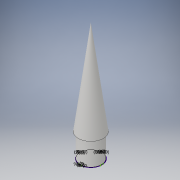
# Autodesk Inventor part: Nose Cone MK II [incomplete]
Saved by Autodesk Inventor 2017 (Build 210142000, 142)
## iProperties
Created: 2017-05-18
Part Number: Nose Cone MK II [incomplete]
Material: Generic
Document SubType Name: Modeling
Designer: Harrison
Density: 1 g/cm^3
Appearance: Default
Author: Harrison
Autodesk Inventor part; units mm, degrees
ref_plane "YZ Plane" through (0, 0, 0) normal (1, 0, 0) x (0, 1, 0)
ref_plane "XZ Plane" through (0, 0, 0) normal (0, 1, 0) x (-1, 0, 0)
ref_plane "XY Plane" through (0, 0, 0) normal (0, 0, 1) x (1, 0, 0)
sketch "Sketch1" plane through (0, 0, 0) normal (1, 0, 0) x (0, 1, 0)
  line L0 (0, 0) -> (101.6, 0)
  line L1 (0, -11.557) -> (0, -13.462)
  line L2 (0, -13.462) -> (101.6, 0)
  line L3 (0, 0) -> (-25.4, 0)
  line L4 (-25.4, 0) -> (-25.4, -11.557)
  line L5 (-25.4, -11.557) -> (0, -11.557)
  line L6 (1.27, -10.287) -> (1.27, -12.0126)
  line L7 (1.27, -12.0126) -> (82.3464, -1.27)
  line L8 (0, -10.287) -> (-24.13, -10.287)
  line L9 (82.3464, -1.27) -> (91.9313, 0)
  line L10 (0, -10.287) -> (1.27, -10.287)
  line L11 (-24.13, -10.287) -> (-25.4, -10.287)
  dimension "d0" = 101.6
  dimension "d1" = 13.462
  dimension "d2" = 25.4
  dimension "d3" = 11.557
  dimension "d4" = 1.27
  dimension "d5" = 1.27
  constraints: 24 end point, 3 perpendicular, 2 horizontal, 2 point on line, 2 vertical
  measures "d0" distance of L0.start L0.end
  measures "d1" distance of L0.start L1.end
  measures "d2" distance of L0.start L3.end
  measures "d3" distance of L3.end L4.end
  measures "d4" distance between parallel lines of L2 L7
  measures "d5" distance between parallel lines of L5 L8
revolve "Revolution1" add sketch "Sketch1" angle 360 about axis through (0, 0, 0) along (0, 1, 0) contours L0 L2 L1 L5 L4 L11 L8 L10 L6 L7 L9
sketch "Sketch2" plane through (0, -25.4, 0) normal (0, -1, 0) x (1, 0, 0)
  circle A0 centre (0, 0) radius 11.557
  circle A1 centre (0, 0) radius 11.811
  circle A2 centre (0, 0) radius 11.557 projected
  line L0 (-0.0952, -11.5566) -> (-1.6827, -11.5566)
  line L1 (-1.6827, -11.5566) -> (1.4923, -11.5566)
  line L2 (-1.6827, -11.5566) -> (1.4923, -11.5566) construction
  line L3 (0, 0) -> (-15.1978, 0)
  line L4 (-11.557, 0) -> (-11.557, -1.5875)
  line L5 (-11.557, 0) -> (-9.9695, 0) construction
  line L6 (-11.557, 0) -> (-11.557, 1.5875)
  line L7 (-0.0029, 11.557) -> (-1.5904, 11.557)
  line L8 (-0.0029, 11.557) -> (1.5846, 11.557)
  line L9 (11.557, -0.0003) -> (11.557, 1.5872)
  line L10 (11.557, -0.0003) -> (13.1445, -0.0003) construction
  line L11 (11.557, 1.5872) -> (11.557, -1.5806)
  line L12 (1.5846, 11.7042) -> (1.5846, 11.4479)
  line L13 (1.5846, 11.7042) -> (1.8409, 11.7042) construction
  line L14 (-1.5846, 11.7042) -> (-1.5846, 11.4479)
  line L15 (-1.5846, 11.7042) -> (-1.3282, 11.7042) construction
  line L16 (-11.4484, 1.5806) -> (-11.7048, 1.5806)
  line L17 (-11.7048, -1.5806) -> (-11.4474, -1.5882)
  line L18 (11.7048, -1.5806) -> (11.4484, -1.5806)
  circle A3 centre (0, 0) radius 11.557
  circle A4 centre (0, 0) radius 11.811
  line L19 (-11.7042, -1.5846) -> (-11.4479, -1.5846)
  line L20 (-11.7042, -1.5846) -> (-11.7042, -1.3282) construction
  line L21 (-11.557, -0.0029) -> (-11.557, -1.5904)
  line L22 (-11.557, -0.0029) -> (-11.557, 1.5846)
  line L23 (-11.7042, 1.5846) -> (-11.4479, 1.5846)
  line L24 (-11.7042, 1.5846) -> (-11.7042, 1.8409) construction
  circle A5 centre (0, 0) radius 11.557
  circle A6 centre (0, 0) radius 11.811
  line L25 (1.5846, -11.7042) -> (1.5846, -11.4479)
  line L26 (1.5846, -11.7042) -> (1.3282, -11.7042) construction
  line L27 (0.0029, -11.557) -> (1.5904, -11.557)
  line L28 (0.0029, -11.557) -> (-1.5846, -11.557)
  line L29 (-1.5846, -11.7042) -> (-1.5846, -11.4479)
  line L30 (-1.5846, -11.7042) -> (-1.8409, -11.7042) construction
  circle A7 centre (0, 0) radius 11.557
  circle A8 centre (0, 0) radius 11.811
  line L31 (11.7042, 1.5846) -> (11.4479, 1.5846)
  line L32 (11.7042, 1.5846) -> (11.7042, 1.3282) construction
  line L33 (11.557, 0.0029) -> (11.557, 1.5904)
  line L34 (11.557, 0.0029) -> (11.557, -1.5846)
  line L35 (11.7042, -1.5846) -> (11.4479, -1.5846)
  line L36 (11.7042, -1.5846) -> (11.7042, -1.8409) construction
  point P0 (11.5566, -0.0952)
  point P1 (0.0003, 11.557)
  point P2 (-1.5806, -11.4484)
  point P3 (1.5882, -11.4474)
  point P4 (-1.5806, -11.7048)
  point P5 (1.5806, -11.7048)
  point P6 (1.5806, 11.7048)
  point P7 (0.0952, 11.5566)
  point P8 (-11.557, 0.0003)
  point P9 (11.4484, -1.5806)
  point P10 (11.4474, 1.5882)
  point P11 (11.7048, -1.5806)
  point P12 (11.7048, 1.5806)
  point P13 (-11.7048, 1.5806)
  point P14 (-11.5566, 0.0952)
  point P15 (-0.0003, -11.557)
  point P16 (1.5806, 11.4484)
  point P17 (-1.5882, 11.4474)
  point P18 (1.5806, 11.7048)
  point P19 (-1.5806, 11.7048)
  point P20 (-1.5806, -11.7048)
  dimension "d7" = 0.254
  dimension "d8" = 1.5875
  dimension "d9" = 3.175
  dimension "d10" = 0
  dimension "d11" = 1.5875
  dimension "d12" = 90
  dimension "d13" = 1.5875
  dimension "d14" = 1.5875
  dimension "d15" = 1.5875
  dimension "d20" = 90
  dimension "d21" = 90
  dimension "d25" = 360
  constraints: 74 end point, 40 point on circle, 10 horizontal, 8 centre point, 6 point on line, 5 equal length, 2 perpendicular, 2 vertical, 1 coincident, 1 collinear, 1 tangent, 111 other
  measures "d7" radial gap between concentric circles of A0 A1
  measures "d8" distance of L0.start L0.end
  measures "d9" distance of L0.end L1.end
  measures "d10" distance between parallel lines of L1 L2
  measures "d11" distance of L4.start L4.end
  measures "d12" angle of L4 L5
  measures "d13" distance of L4.start L6.end
  measures "d14" distance of L7.start L7.end
  measures "d15" distance of L7.start L8.end
  measures "d20" angle of L12 L13
  measures "d21" angle of L14 L15
body "Solid1"
